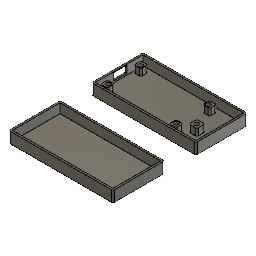
ElektronikTmpNow (Autodesk Fusion 360 design; units mm, degrees)
Autodesk Fusion 360 part; units mm, degrees
sketch "Skizze1" plane through (0, 0, 0) normal (0, 1, 0) x (1, 0, 0)
  line L0 (0, 0) -> (48, 0)
  line L1 (48, 0) -> (48, -25.5)
  line L2 (48, -25.5) -> (0, -25.5)
  line L3 (0, -25.5) -> (0, 0)
  circle A0 centre (45.5, -2.5) radius 1.4
  line L4 (24, 5) -> (24, -28) construction
  line L5 (-2.2203, -12.75) -> (51, -12.75) construction
  circle A1 centre (45.5, -23) radius 1.4
  circle A2 centre (2.5, -2.5) radius 1.4
  circle A3 centre (2.5, -23) radius 1.4
  line L6 (50, -6) -> (60.5, -6)
  line L7 (60.5, -6) -> (60.5, -19.5)
  line L8 (60.5, -19.5) -> (50, -19.5)
  line L9 (50, -19.5) -> (50, -6)
  circle A4 centre (52.5, -17) radius 1.4
  line L10 (-1, 2.4) -> (62.9, 2.4)
  line L11 (62.9, 2.4) -> (62.9, -27.9)
  line L12 (62.9, -27.9) -> (-1, -27.9)
  line L13 (-1, -27.9) -> (-1, 2.4)
  line L14 (64.1, 3.6) -> (64.1, -29.1)
  line L15 (64.1, -29.1) -> (-2.2, -29.1)
  line L16 (-2.2, -29.1) -> (-2.2, 3.6)
  line L17 (-2.2, 3.6) -> (64.1, 3.6)
  line L18 (48, -4.3) -> (43.7, -4.3)
  line L19 (43.7, -4.3) -> (43.7, 0)
  line L20 (43.7, -21.2) -> (43.7, -25.5)
  line L21 (48, -21.2) -> (43.7, -21.2)
  line L22 (0, -4.3) -> (4.3, -4.3)
  line L23 (4.3, -4.3) -> (4.3, 0)
  line L24 (0, -21.2) -> (4.3, -21.2)
  line L25 (4.3, -21.2) -> (4.3, -25.5)
  line L26 (50, -14.4) -> (55.1, -14.4)
  line L27 (55.1, -14.4) -> (55.1, -19.5)
  line L28 (-2.2, -49.1) -> (64.1, -49.1)
  line L29 (64.1, -49.1) -> (64.1, -81.8)
  line L30 (64.1, -81.8) -> (-2.2, -81.8)
  line L31 (-2.2, -81.8) -> (-2.2, -49.1)
  line L32 (62.9, -80.6) -> (-1, -80.6)
  line L33 (-1, -80.6) -> (-1, -50.3)
  line L34 (-1, -50.3) -> (62.9, -50.3)
  line L35 (62.9, -50.3) -> (62.9, -80.6)
  dimension "d1" = 48
  dimension "d2" = 25.5
  dimension "d3" = 2.8
  dimension "d4" = 2.5
  dimension "d5" = 2.5
  dimension "d6" = 24
  dimension "d7" = 12.75
  dimension "d8" = 13.5
  dimension "d9" = 10.5
  dimension "d10" = 2.8
  dimension "d11" = 2.5
  dimension "d12" = 2.5
  dimension "d13" = 6
  dimension "d14" = 2
  dimension "d15" = 1
  dimension "d16" = 2.4
  dimension "d17" = 2.4
  dimension "d18" = 2.4
  dimension "d19" = -1.2
  dimension "d20" = 4.3
  dimension "d21" = 4.3
  dimension "d22" = 5.1
  dimension "d24" = 5.1
  dimension "d41" = 67.7
  dimension "d42" = 32.7
  dimension "d44" = 20
  dimension "d45" = 1.2
  constraint horizontal L0
  constraint vertical L1
  constraint horizontal L2
  constraint vertical L3
  constraint coincident L0.start L3.end
  constraint perpendicular L2 L4
  constraint perpendicular L1 L5
  constraint symmetric A0 L5 A1
  constraint symmetric A0 L4 A2
  constraint symmetric L4 A1 A3
  constraint horizontal L6
  constraint vertical L7
  constraint horizontal L8
  constraint vertical L9
  constraint horizontal L10
  constraint vertical L11
  constraint horizontal L12
  constraint vertical L13
  constraint coincident L1 L18.start
  constraint perpendicular L1 L18
  constraint coincident L0 L19.end
  constraint perpendicular L0 L19
  constraint symmetric L5 L18.start L21.start
  constraint symmetric L5 L18.end L20.start
  constraint symmetric L5 L19.end L20.end
  constraint symmetric L4 L18.start L22.start
  constraint symmetric L4 L18.end L22.end
  constraint symmetric L4 L19.end L23.end
  constraint symmetric L4 L20.start L24.end
  constraint symmetric L4 L20.end L25.end
  constraint symmetric L4 L21.start L24.start
  constraint coincident L9 L26.start
  constraint perpendicular L9 L26
  constraint coincident L8 L27.end
  constraint perpendicular L8 L27
  constraint horizontal L28
  constraint vertical L29
  constraint horizontal L30
  constraint vertical L31
  constraint collinear L14 L29
  constraint equal L15 L28
  constraint equal L16 L31
  measures "d1" distance of L0.start L0.end
  measures "d2" distance of L0.start L2.end
  measures "d3" diameter of A0
  measures "d4" distance of L0 A0.centre
  measures "d5" distance of L1 A0.centre
  measures "d6" distance of L3 L4
  measures "d7" distance of L2 L5
  measures "d8" distance of L6.start L8.end
  measures "d9" distance of L6.start L6.end
  measures "d10" diameter of A4
  measures "d11" distance of L9 A4.centre
  measures "d12" distance of L8 A4.centre
  measures "d13" distance of L0 L6
  measures "d14" distance of L1 L9 L0.start
  measures "d15" distance of L3 L13
  measures "d16" distance of L0 L10
  measures "d17" distance of L2 L12
  measures "d18" distance of L7 L11
  measures "d20" distance of L1 L19
  measures "d21" distance of L0 L18
  measures "d22" distance of L9 L27
  measures "d24" distance of L8 L26
  measures "d42" distance of L15.end L16.end
  measures "d44" distance of L15 L28
extrude "Extrusion1" add sketch "Skizze1" along normal blind 1 contours L0 L3 L22 L23 | L0 L1 L2 L3 L18 L19 L20 L21 L22 L23 L24 L25 | L0 L1 L18 L19 | L2 L3 L24 L25 | L1 L2 L20 L21 | A0 | A1 | A2 | A3 | L6 L7 L8 L9 L26 L27 | L8 L9 L26 L27 | A4 | L10 L11 L12 L13 | L14 L15 L16 L17 | L28 L29 L30 L31 | L32 L33 L34 L35 makes body 1 at (19.9, 0, 18.2) makes body 2 at (19.9, 0, 60)
extrude "Extrusion2" add sketch "Skizze1" along normal blind 7 contours L14 L15 L16 L17 bodies 1
extrude "Extrusion3" add sketch "Skizze1" along normal blind 5.4 contours L0 L3 L22 L23 | L0 L1 L18 L19 | L2 L3 L24 L25 | L1 L2 L20 L21 | L8 L9 L26 L27 bodies 1
sketch "Skizze2" plane through (-2.2, 0, 0) normal (-1, 0, 0) x (0, 0, 1)
  line L0 (-3.6, 0) -> (29.1, 0)
  line L1 (29.1, 0) -> (29.1, 7)
  line L2 (29.1, 7) -> (-3.6, 7)
  line L3 (-3.6, 7) -> (-3.6, 0)
  line L4 (7.75, 6.4) -> (16.15, 6.4)
  line L5 (16.15, 6.4) -> (16.15, 2)
  line L6 (16.15, 2) -> (7.75, 2)
  line L7 (7.75, 2) -> (7.75, 6.4)
  line L8 (29.1, 0) -> (-3.6, 0)
  dimension "d31" = 8.4
  dimension "d32" = 4.4
  dimension "d34" = 2
  dimension "d35" = 34.3
  dimension "d36" = 12.95
  constraint horizontal L4
  constraint vertical L5
  constraint horizontal L6
  constraint vertical L7
  measures "d31" distance of L4.start L4.end
  measures "d32" distance of L4.start L6.end
  measures "d34" distance of L6 L8
  measures "d36" distance of L1 L5
extrude "Extrusion4" cut sketch "Skizze2" against normal up to surface (1.2 mm away) contours L4 L5 L6 L7 bodies 1
extrude "Extrude5" add sketch "Skizze1" along normal blind 7 contours L28 L29 L30 L31 bodies 2
fillet "Abrundung1" radius 1 24 edges at (64.1, 3.5, -3.6) (-2.2, 3.5, -3.6) (0, 3.2, 0) (4.3, 3.2, 0) (43.7, 3.2, 0) (48, 3.2, 0) (50, 3.2, 14.4) (55.1, 3.2, 14.4) (48, 3.2, 21.2) (43.7, 3.2, 21.2) (4.3, 3.2, 21.2) (0, 3.2, 21.2) (-2.2, 3.5, 29.1) (64.1, 3.5, 29.1) (55.1, 3.2, 19.5) (50, 3.2, 19.5) (48, 3.2, 25.5) (43.7, 3.2, 25.5) (4.3, 3.2, 25.5) (0, 3.2, 25.5) (4.3, 3.2, 4.3) (0, 3.2, 4.3) (43.7, 3.2, 4.3) (48, 3.2, 4.3) on bodies 1 2
fillet "Abrundung1" radius 1 4 edges at (-2.2, 3.5, 81.8) (-2.2, 3.5, 49.1) (64.1, 3.5, 81.8) (64.1, 3.5, 49.1) on bodies 1 2
equation "d6 = d1 / 2"
equation "d7 = d2 / 2"
equation "d13 = ( d2 - d8 ) / 2"
equation "d20 = d5 + d3 / 2 + 0.4 mm"
equation "d21 = d20"
equation "d22 = d11 + d10 / 2 + 1.2 mm"
equation "d24 = d22"
equation "d36 = ( 34.30 mm - d31 ) / 2"
